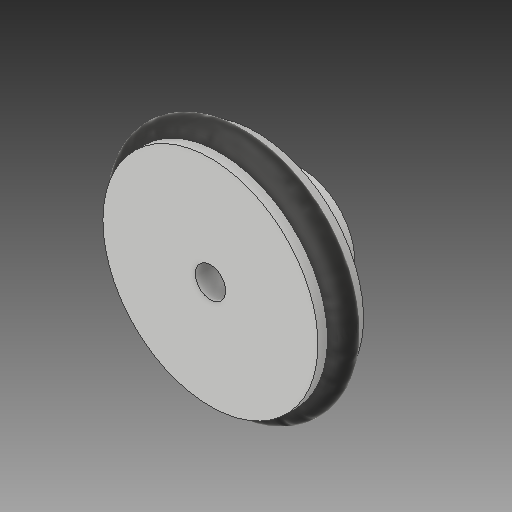
# Autodesk Inventor part: Roue de mesure Scancon 100 mm -ID64
Saved by Autodesk Inventor 2017 (Build 210142000, 142)
## iProperties
Created: 2017-12-17
Part Number: Roue de mesure Scancon 100 mm -ID64
Material: Generic
Document SubType Name: Modeling
Designer: Aegir
Density: 1 g/cm^3
Appearance: Default
Mass: 5.00554 g
Surface Area: 24.0056 cm^2
Volume: 5.00554 cm^3
Author: Aegir
Autodesk Inventor part; units mm, degrees
ref_plane "YZ Plane" through (0, 0, 0) normal (1, 0, 0) x (0, 1, 0)
ref_plane "XZ Plane" through (0, 0, 0) normal (0, 1, 0) x (-1, 0, 0)
ref_plane "XY Plane" through (0, 0, 0) normal (0, 0, 1) x (1, 0, 0)
sketch "Esquisse1" plane through (0, 0, 0) normal (0, 1, 0) x (-1, 0, 0)
  line L0 (2.6673, 3.1855) -> (14.165, 3.1855)
  line L1 (14.165, 3.1855) -> (14.165, 1.9355)
  line L2 (14.165, -1.5645) -> (14.165, -2.8145)
  line L3 (14.165, -2.8145) -> (7, -2.8145)
  line L4 (7, -2.8145) -> (7, -8.8145)
  line L5 (7, -8.8145) -> (2, -8.8145)
  line L6 (2, -8.8145) -> (2, 3.1855)
  line L7 (2, 3.1855) -> (2.6673, 3.1855)
  line L8 (0, -11.2145) -> (0, 5.5855) projected
  arc A0 (14.165, -1.5645) -> (14.165, 1.9355) centre (14.165, 0.1855) ccw
  point P0 (0, 0)
  dimension "d0" = 12
  dimension "d2" = 6
  dimension "d4" = 2
  dimension "d5" = 7
  dimension "d8" = 14.165
  dimension "d10" = 14.165
  dimension "d11" = 3
  dimension "d12" = 1.75
  constraints: 16 end point, 6 perpendicular, 2 point on circle, 1 centre point, 1 horizontal, 1 vertical
  measures "d0" distance between parallel lines of L0 L5
  measures "d2" distance between parallel lines of L3 L0
  measures "d4" distance from line of L6 point (0, 0)
  measures "d5" distance from line of L4 point (0, 0)
  measures "d8" horizontal distance of A0.centre point (0, 0)
  measures "d10" distance between parallel lines of L8 L2
  measures "d11" distance from line of L0 A0.centre
  measures "d12" radius of A0
revolve "Révolution1" add sketch "Esquisse1" angle 360 about axis through (0, 0, -10) along (0, 0, 1)
